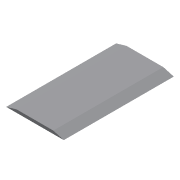
# Autodesk Inventor part: two sides with ramps
Saved by Autodesk Inventor 2015 (Build 190159000, 159)
## iProperties
Created: 2015-01-03
Part Number: two sides with ramps
Material: Generic
Document SubType Name: Modeling
Designer: Peter
Density: 1 g/cm^3
Appearance: Default
Author: Peter
Autodesk Inventor part; units mm, degrees
ref_plane "YZ Plane" through (0, 0, 0) normal (1, 0, 0) x (0, 1, 0)
ref_plane "XZ Plane" through (0, 0, 0) normal (0, 1, 0) x (-1, 0, 0)
ref_plane "XY Plane" through (0, 0, 0) normal (0, 0, 1) x (1, 0, 0)
sketch "Sketch1" plane through (0, 0, 0) normal (0, 0, 1) x (1, 0, 0)
  line L0 (0, 0) -> (173.9643, 49.8835)
  line L1 (173.9643, 49.8835) -> (783.5643, 49.8835)
  line L2 (783.5643, 49.8835) -> (957.5287, 0)
  line L3 (957.5287, 0) -> (0, 0)
  dimension "incline" = 180.975
  dimension "Width" = 609.6
  dimension "d2" = 49.8835
  dimension "angle" = 16
  constraints: 8 end point, 1 equal length, 1 horizontal, 1 parallel
  measures "incline" distance of L0.start L0.end
  measures "Width" distance of L0.end L1.end
  measures "d2" vertical distance of L0.start L0.end
  measures "angle" angle of L3 L2
extrude "Extrusion1" add sketch "Sketch1" along normal blind 1828.8
body "Solid1"
